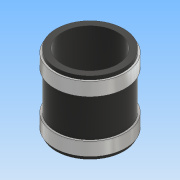
# Autodesk Inventor part: 4082
Saved by Autodesk Inventor 2018.1 (Build 221171000, 171)
## iProperties
Created: 2019-03-20
Part Number: 4082
Material: PVC-Piping
Document SubType Name: Modeling
Designer: James
Density: 1.4 g/cm^3
Appearance: Smooth - Black
Description: 42-50mm EPDM Adaptor
Author: James
Autodesk Inventor part; units mm, degrees
ref_plane "YZ Plane" through (0, 0, 0) normal (1, 0, 0) x (0, 1, 0)
ref_plane "XZ Plane" through (0, 0, 0) normal (0, 1, 0) x (-1, 0, 0)
ref_plane "XY Plane" through (0, 0, 0) normal (0, 0, 1) x (1, 0, 0)
sketch "Sketch1" plane through (0, 0, 0) normal (0, 0, 1) x (1, 0, 0)
  circle A0 centre (0, 0) radius 23
  circle A1 centre (0, 0) radius 28
  dimension "d0" = 46
  dimension "d1" = 56
  constraints: 2 centre point, 2 coincident
  measures "d0" diameter of A0
  measures "d1" diameter of A1
extrude "Extrusion1" add sketch "Sketch1" along normal mid plane 60
sketch "Sketch2" plane through (0, 0, 0) normal (1, 0, 0) x (0, 1, 0)
  line L0 (28, 27) -> (29.5, 27)
  line L1 (29.5, 27) -> (29.5, 16)
  line L2 (29.5, 16) -> (28, 16)
  line L3 (28, 16) -> (28, 27)
  line L4 (28, -16) -> (29.5, -16)
  line L5 (29.5, -16) -> (29.5, -27)
  line L6 (29.5, -27) -> (28, -27)
  line L7 (28, -27) -> (28, -16)
  line L8 (28, 30) -> (-28, 30) projected
  line L9 (-28, -30) -> (28, -30) projected
  line L10 (0, -42) -> (0, 42) projected
  point P0 (0, 0)
  dimension "d4" = 1.5
  dimension "d5" = 11
  dimension "d6" = 3
  dimension "d7" = 3
  dimension "d8" = 11
  constraints: 16 end point, 4 parallel, 2 horizontal, 2 perpendicular, 2 point on line, 2 vertical alignment
  measures "d4" distance of L0.start L0.end
  measures "d5" distance of L0.end L1.end
  measures "d6" distance from line of L0 L8.start
  measures "d7" distance between parallel lines of L9 L6
  measures "d8" distance of L4.end L5.end
revolve "Revolution1" add sketch "Sketch2" angle 360 about axis through (0, 0, -10) along (0, 0, 1)
equation "\"d7\" = d6"
equation "\"d8\" = d5"
body "Solid1"
